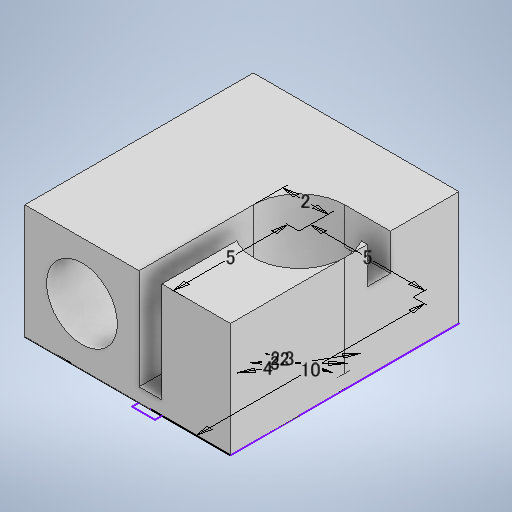
# Autodesk Inventor part: rod4.3
Saved by Autodesk Inventor 2025 (Build 290162000, 162)
## iProperties
Created: 2024-07-13
Part Number: rod4.3
Material: 一般
Document SubType Name: Modeling
Designer: Saigusa
Density: 1 g/cm^3
Appearance: 既定
Author: Saigusa
Autodesk Inventor part; units mm, degrees
ref_plane "YZ Plane" through (0, 0, 0) normal (1, 0, 0) x (0, 1, 0)
ref_plane "XZ Plane" through (0, 0, 0) normal (0, 1, 0) x (-1, 0, 0)
ref_plane "XY Plane" through (0, 0, 0) normal (0, 0, 1) x (1, 0, 0)
sketch "スケッチ1" plane through (0, 0, 0) normal (0, 1, 0) x (-1, 0, 0)
  circle A0 centre (0, 0) radius 1.15
  circle A1 centre (0, 0) radius 1
  circle A2 centre (0, 0) radius 1.5
  circle A3 centre (0, 0) radius 2
  line L0 (1.5, 0) -> (1, 0)
  line L1 (1, 0) -> (1, 2)
  line L2 (1, 2) -> (1.5, 2)
  line L3 (1.5, 2) -> (1.5, 0)
  line L4 (0, 0) -> (5, 0)
  line L5 (5, 0) -> (5, -5)
  line L6 (5, -5) -> (0, -5)
  line L7 (0, -5) -> (0, 0)
  line L8 (5, -5) -> (0, -5)
  line L9 (0, -5) -> (0, 5)
  line L10 (0, 5) -> (5, 5)
  line L11 (5, 5) -> (5, -5)
  line L12 (0, 0) -> (-2, 0)
  line L13 (-2, 0) -> (-2, -5)
  line L14 (-2, -5) -> (0, -5)
  line L15 (0, -5) -> (0, 0)
  line L16 (-2, -5) -> (1.5, -5)
  line L17 (1.5, -5) -> (1.5, -1.5)
  line L18 (1.5, -1.5) -> (-2, -1.5)
  line L19 (-2, -1.5) -> (-2, -5)
  line L20 (1.5, 2) -> (-2, 2)
  line L21 (-2, 2) -> (-2, 5)
  line L22 (-2, 5) -> (1.5, 5)
  line L23 (1.5, 5) -> (1.5, 2)
  line L24 (-2, 2) -> (1.5, 2)
  line L25 (1.5, 2) -> (1.5, -1.5)
  line L26 (1.5, -1.5) -> (-2, -1.5)
  line L27 (-2, -1.5) -> (-2, 2)
  line L28 (0, -1) -> (-2, -1)
  line L29 (1.5, 2) -> (1, 2)
  line L30 (1, 2) -> (1, 5)
  line L31 (1, 5) -> (1.5, 5)
  line L32 (1.5, 5) -> (1.5, 2)
  line L33 (5, 5) -> (7, 5)
  line L34 (7, 5) -> (7, -5)
  line L35 (7, -5) -> (5, -5)
  line L36 (5, -5) -> (5, 5)
  line L37 (1, 0) -> (2, 0)
  line L38 (2, 0) -> (2, 5.3047)
  line L39 (2, 5.3047) -> (1, 5.3047)
  line L40 (1, 5.3047) -> (1, 0)
  line L41 (0, -2) -> (-2, -2)
  line L42 (-2, -2) -> (-2, -1)
  line L43 (-2, -1) -> (0, -1)
  line L44 (0, -1) -> (0, -2)
  point P0 (0, -1.5)
  point P1 (-2, -1.5)
  point P2 (0, 2)
  point P3 (1, 1.118)
  point P4 (-1.118, -1)
  point P5 (1.5, 5)
  point P6 (1, 1.7321)
  point P7 (-1.7321, -1)
  point P8 (2, 5)
  dimension "d2" = 3
  dimension "d3" = 4
  dimension "d0" = 2.3
  dimension "d1" = 2
  dimension "d4" = 5
  dimension "d5" = 5
  dimension "d6" = 10
  dimension "d15" = 2
  constraints: 90 end point, 22 parallel, 12 perpendicular, 11 horizontal, 11 point on line, 4 coincident, 2 centre point, 2 point on circle, 1 tangent, 6 other
  measures "d0" diameter of A0
  measures "d1" diameter of A1
  measures "d4" distance of L5.end L6.end
  measures "d5" distance of L4.end L5.end
  measures "d6" distance of L8.end L9.end
  measures "d15" distance of L34.end L35.end
extrude "押し出し1" add sketch "スケッチ1" along normal blind 5 contours L4 L5 L6 L17 L25 A3 | L38 L10 L11 L4 | L25 L18 A3 | A3 L20 L1 | A3 L18 L17 L6 L7 | L7 L14 L13 L41 | L11 L33 L34 L35 L5 | L20 L21 L22 L9 | L9 L10 L30 L20 | A3 L27 L20 | L28 L13 A3
extrude "押し出し2" add sketch "スケッチ1" along normal blind 0.6 contours L0 L1 A0 | L0 A2 L7 A0 | A0 L1 A2 L0 | A0 L7 A1 L0 | L1 A1 L9 A0 | A0 L9 A2 L1 | L7 A2 L28 A0 | A0 L28 L7 | L25 A3 L18 A2 | A2 L1 A3 L3 | L3 A3 L4 | L4 A3 L25 | L9 A1 L12 A0 | A0 L12 A2 L9 | A2 L9 A3 L1 | L28 A2 L12 A0 | A0 L12 A1 L28 | L18 A3 L28 A2 | L18 A3 L7 | L7 A3 L18 | L3 L23 L10 L38 A3 | A3 L1 L2 L3 | A2 L12 A3 L9 | L28 A3 L12 A2 | L41 L13 L18 A3 | L18 L13 L28 A3 | L2 L30 L10 L23
extrude "押し出し4" add sketch "スケッチ1" along normal blind 3.4 contours L41 L13 L18 A3 | L18 L13 L28 A3
sketch "スケッチ4" plane through (-7, 0, 5) normal (0, 0, 1) x (1, 0, 0)
  line L0 (9, 5) -> (0, 5) projected
  line L1 (0, 5) -> (2.5, 5)
  line L2 (2.5, 5) -> (2.5, 2.5)
  line L3 (2.5, 2.5) -> (0, 2.5)
  line L4 (0, 2.5) -> (0, 5)
  point P0 (7, 0)
  dimension "d25" = 2.5
  dimension "d26" = 2.5
  constraints: 8 end point, 2 parallel, 1 horizontal, 1 perpendicular
  measures "d25" distance of L2.end L3.end
  measures "d26" distance of L1.end L2.end
hole "穴2" at (-4.5, 2.5, 5) direction (0, 0, -1) diameter 3.1 depth 8
